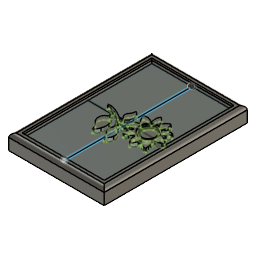
Test 2 tournesol (Autodesk Fusion 360 design; units mm, degrees)
part number: 2026-04-24-15-50-29-841
Autodesk Fusion 360 part; units mm, degrees
box "BoitePrimitive1" add length 75 width 50 height 8 placed x (0, -1, 0) y (1, 0, 0) z (0, 0, 1) at (0, 0, 0)
sketch "Esquisse2" plane through (0, 0, 8) normal (0, 0, 1) x (-1, 0, 0)
  line L0 (0, 75) -> (-50, 75)
  line L1 (-50, 75) -> (-50, 0)
  line L2 (-50, 0) -> (0, 0)
  line L3 (0, 0) -> (0, 75)
  line L4 (-4.0213, 75) -> (-4.0213, 0)
  line L5 (0, 4.0248) -> (-50, 4.0248)
  line L6 (-46.0257, 0) -> (-46.0257, 75)
  line L7 (-50, 70.9503) -> (0, 70.9503)
  point P0 (-4.0213, 70.9503)
  point P1 (-46.0257, 70.9503)
  point P2 (-46.0257, 4.0248)
  point P3 (-4.0213, 4.0248)
  constraint coincident L0 L4.start
  constraint coincident L2 L4.end
  constraint perpendicular L2 L4
  constraint coincident L3 L5.start
  constraint coincident L1 L5.end
  constraint perpendicular L1 L5
  constraint coincident L2 L6.start
  constraint coincident L0 L6.end
  constraint perpendicular L0 L6
  constraint coincident L1 L7.start
  constraint coincident L3 L7.end
  constraint perpendicular L3 L7
  constraint coincident L7 P0
  constraint coincident L4 P0
  constraint coincident L6 P1
  constraint coincident L7 P1
  constraint coincident L6 P2
  constraint coincident L5 P2
  constraint coincident L5 P3
  constraint coincident L4 P3
extrude "Extrusion1" cut sketch "Esquisse2" against normal blind 2 contours L4 L5 L6 L7
fillet "Congé1" radius 2 4 edges at (25, 0, 8) (50, -37.5, 8) (25, -75, 8) (0, -37.5, 8)
fillet "Congé2" radius 0.5 4 edges at (25.0235, -4.0248, 8) (46.0257, -37.4876, 8) (25.0235, -70.9503, 8) (4.0213, -37.4876, 8)
sketch "Esquisse3" plane through (0, 0, 6) normal (0, 0, 1) x (-1, 0, 0)
  line L0 (-46.0257, 4.0248) -> (-4.0213, 4.0248)
  line L1 (-4.0213, 4.0248) -> (-4.0213, 70.9503)
  line L2 (-4.0213, 70.9503) -> (-46.0257, 70.9503)
  line L3 (-46.0257, 70.9503) -> (-46.0257, 4.0248)
  line L4 (-25.0235, 4.0248) -> (-25.0235, 70.9503)
  line L5 (-4.0213, 37.4876) -> (-46.0257, 37.4876)
  line L6 (-25.4937, 4.0248) -> (-25.4937, 70.9503)
  line L7 (-24.5013, 4.0248) -> (-24.5013, 70.9503)
  spline S0 degree 3 poles (-13.2534, 35.811) (-13.4823, 35.5969) (-15.4305, 35.9038) (-16.7842, 36.3672) knots 0 0 0 0 1 1 1 1
  spline S1 degree 3 poles (-16.7842, 36.3672) (-17.692, 36.678) (-19.587, 37.5732) (-20.54, 38.1415) knots 0 0 0 0 1 1 1 1
  spline S2 degree 3 poles (-20.54, 38.1415) (-21.6835, 38.8234) (-22.4957, 39.02) (-23.1364, 38.7701) knots 0 0 0 0 1 1 1 1
  spline S3 degree 3 poles (-23.1364, 38.7701) (-23.4033, 38.666) (-23.4058, 38.6626) (-23.3252, 38.5087) knots 0 0 0 0 1 1 1 1
  spline S4 degree 3 poles (-23.3252, 38.5087) (-23.2804, 38.4229) (-23.0386, 38.1071) (-22.7879, 37.807) knots 0 0 0 0 1 1 1 1
  spline S5 degree 3 poles (-22.7879, 37.807) (-22.5373, 37.5068) (-22.2677, 37.1329) (-22.1889, 36.9761) knots 0 0 0 0 1 1 1 1
  spline S6 degree 3 poles (-22.1889, 36.9761) (-21.8625, 36.3265) (-21.9778, 35.5072) (-22.4877, 34.8523) knots 0 0 0 0 1 1 1 1
  spline S7 degree 3 poles (-22.4877, 34.8523) (-23.2739, 33.8426) (-23.3292, 33.7283) (-23.4429, 32.8776) knots 0 0 0 0 1 1 1 1
  spline S8 degree 3 poles (-23.4429, 32.8776) (-23.5405, 32.1474) (-23.5565, 32.0964) (-23.7039, 32.0427) knots 0 0 0 0 1 1 1 1
  spline S9 degree 3 poles (-23.7039, 32.0427) (-23.8507, 31.9893) (-23.8907, 32.0077) (-24.3137, 32.3228) knots 0 0 0 0 1 1 1 1
  spline S10 degree 3 poles (-24.3137, 32.3228) (-25.4296, 33.1541) (-26.1693, 34.5636) (-26.1594, 35.8399) knots 0 0 0 0 1 1 1 1
  spline S11 degree 3 poles (-26.1594, 35.8399) (-26.1548, 36.4262) (-25.9675, 37.136) (-25.7116, 37.5369) knots 0 0 0 0 1 1 1 1
  spline S12 degree 3 poles (-25.7116, 37.5369) (-25.4079, 38.0125) (-24.7673, 38.5558) (-24.2808, 38.7503) knots 0 0 0 0 1 1 1 1
  spline S13 degree 3 poles (-24.2808, 38.7503) (-24.0446, 38.8447) (-23.717, 39) (-23.5527, 39.0955) knots 0 0 0 0 1 1 1 1
  spline S14 degree 3 poles (-23.5527, 39.0955) (-23.1919, 39.3052) (-22.7265, 39.3936) (-22.2525, 39.3422) knots 0 0 0 0 1 1 1 1
  spline S15 degree 3 poles (-22.2525, 39.3422) (-22.0589, 39.3212) (-21.9143, 39.3361) (-21.9312, 39.3753) knots 0 0 0 0 1 1 1 1
  spline S16 degree 3 poles (-21.9312, 39.3753) (-22.0154, 39.5708) (-23.3025, 40.3477) (-24.3294, 40.823) knots 0 0 0 0 1 1 1 1
  spline S17 degree 3 poles (-24.3294, 40.823) (-25.2456, 41.2471) (-25.5259, 41.3479) (-26.188, 41.4917) knots 0 0 0 0 1 1 1 1
  spline S18 degree 3 poles (-26.188, 41.4917) (-27.4482, 41.7653) (-28.566, 41.7741) (-29.7633, 41.5197) knots 0 0 0 0 1 1 1 1
  spline S19 degree 3 poles (-29.7633, 41.5197) (-30.0286, 41.4634) (-30.3169, 41.4134) (-30.4041, 41.4085) knots 0 0 0 0 1 1 1 1
  spline S20 degree 3 poles (-30.4041, 41.4085) (-30.609, 41.3973) (-31.0876, 40.728) (-31.0212, 40.5455) knots 0 0 0 0 1 1 1 1
  spline S21 degree 3 poles (-31.0212, 40.5455) (-31.0135, 40.5245) (-30.8196, 40.5139) (-30.5901, 40.522) knots 0 0 0 0 1 1 1 1
  spline S22 degree 3 poles (-30.5901, 40.522) (-30.3607, 40.5301) (-30.1121, 40.5389) (-30.0376, 40.5415) knots 0 0 0 0 1 1 1 1
  spline S23 degree 3 poles (-30.0376, 40.5415) (-29.7942, 40.5502) (-29.0635, 40.4545) (-28.6359, 40.3579) knots 0 0 0 0 1 1 1 1
  spline S24 degree 3 poles (-28.6359, 40.3579) (-28.2014, 40.2597) (-26.5617, 39.5188) (-26.2895, 39.2977) knots 0 0 0 0 1 1 1 1
  spline S25 degree 3 poles (-26.2895, 39.2977) (-26.1466, 39.1816) (-26.1483, 39.1565) (-26.3238, 38.7809) knots 0 0 0 0 1 1 1 1
  spline S26 degree 3 poles (-26.3238, 38.7809) (-26.4253, 38.5638) (-26.5807, 38.3308) (-26.6691, 38.2631) knots 0 0 0 0 1 1 1 1
  spline S27 degree 3 poles (-26.6691, 38.2631) (-26.7575, 38.1954) (-26.8893, 38.0659) (-26.9619, 37.9752) knots 0 0 0 0 1 1 1 1
  spline S28 degree 3 poles (-26.9619, 37.9752) (-27.0345, 37.8846) (-27.2951, 37.6725) (-27.5409, 37.5038) knots 0 0 0 0 1 1 1 1
  spline S29 degree 3 poles (-27.5409, 37.5038) (-27.7867, 37.3352) (-27.9969, 37.1778) (-28.008, 37.154) knots 0 0 0 0 1 1 1 1
  spline S30 degree 3 poles (-28.008, 37.154) (-28.019, 37.1303) (-28.1248, 37.0882) (-28.243, 37.0605) knots 0 0 0 0 1 1 1 1
  spline S31 degree 3 poles (-28.243, 37.0605) (-28.3612, 37.0328) (-28.4608, 36.9866) (-28.4644, 36.9579) knots 0 0 0 0 1 1 1 1
  spline S32 degree 3 poles (-28.4644, 36.9579) (-28.4754, 36.8699) (-29.5329, 36.455) (-30.0799, 36.3241) knots 0 0 0 0 1 1 1 1
  spline S33 degree 3 poles (-30.0799, 36.3241) (-30.6696, 36.1831) (-30.6481, 36.1277) (-29.8052, 35.6164) knots 0 0 0 0 1 1 1 1
  spline S34 degree 3 poles (-29.8052, 35.6164) (-29.5603, 35.4678) (-29.0495, 35.0412) (-29.0277, 34.9671) knots 0 0 0 0 1 1 1 1
  spline S35 degree 3 poles (-29.0277, 34.9671) (-29.0195, 34.9392) (-28.9051, 34.8066) (-28.7734, 34.6724) knots 0 0 0 0 1 1 1 1
  spline S36 degree 3 poles (-28.7734, 34.6724) (-28.6418, 34.5382) (-28.4108, 34.2239) (-28.2601, 33.974) knots 0 0 0 0 1 1 1 1
  spline S37 degree 3 poles (-28.2601, 33.974) (-28.1093, 33.724) (-27.9401, 33.4561) (-27.8839, 33.3787) knots 0 0 0 0 1 1 1 1
  spline S38 degree 3 poles (-27.8839, 33.3787) (-27.726, 33.1609) (-27.3691, 32.205) (-27.3593, 31.9737) knots 0 0 0 0 1 1 1 1
  spline S39 degree 3 poles (-27.3593, 31.9737) (-27.3513, 31.7837) (-27.3694, 31.7607) (-27.5812, 31.6926) knots 0 0 0 0 1 1 1 1
  spline S40 degree 3 poles (-27.5812, 31.6926) (-27.9245, 31.5821) (-28.9894, 31.5368) (-29.0506, 31.6301) knots 0 0 0 0 1 1 1 1
  spline S41 degree 3 poles (-29.0506, 31.6301) (-29.0818, 31.6777) (-29.0997, 31.6761) (-29.0938, 31.6263) knots 0 0 0 0 1 1 1 1
  spline S42 degree 3 poles (-29.0938, 31.6263) (-29.0845, 31.5476) (-29.2191, 31.5418) (-29.7301, 31.5993) knots 0 0 0 0 1 1 1 1
  spline S43 degree 3 poles (-29.7301, 31.5993) (-30.2675, 31.6598) (-31.202, 32.0241) (-31.7872, 32.4011) knots 0 0 0 0 1 1 1 1
  spline S44 degree 3 poles (-31.7872, 32.4011) (-32.3647, 32.7733) (-32.5127, 32.7687) (-32.378, 32.3826) knots 0 0 0 0 1 1 1 1
  spline S45 degree 3 poles (-32.378, 32.3826) (-32.144, 31.7115) (-32.0367, 31.2191) (-32.1072, 31.1394) knots 0 0 0 0 1 1 1 1
  spline S46 degree 3 poles (-32.1072, 31.1394) (-32.1271, 31.1169) (-32.1155, 31.0855) (-32.0814, 31.0695) knots 0 0 0 0 1 1 1 1
  spline S47 degree 3 poles (-32.0814, 31.0695) (-32.0008, 31.032) (-31.9788, 30.42) (-32.0551, 30.3394) knots 0 0 0 0 1 1 1 1
  spline S48 degree 3 poles (-32.0551, 30.3394) (-32.0873, 30.3055) (-32.0912, 30.2083) (-32.0638, 30.1235) knots 0 0 0 0 1 1 1 1
  spline S49 degree 3 poles (-32.0638, 30.1235) (-31.9808, 29.8664) (-32.1499, 29.0508) (-32.402, 28.4923) knots 0 0 0 0 1 1 1 1
  line L8 (-32.402, 28.4923) -> (-32.6368, 27.972)
  line L9 (-32.6368, 27.972) -> (-32.889, 28.0653)
  spline S50 degree 3 poles (-32.889, 28.0653) (-33.5693, 28.3168) (-34.7121, 29.5435) (-35.0582, 30.3936) knots 0 0 0 0 1 1 1 1
  spline S51 degree 3 poles (-35.0582, 30.3936) (-35.1169, 30.5376) (-35.1832, 30.664) (-35.2056, 30.6745) knots 0 0 0 0 1 1 1 1
  spline S52 degree 3 poles (-35.2056, 30.6745) (-35.228, 30.6849) (-35.3089, 30.8654) (-35.3854, 31.0754) knots 0 0 0 0 1 1 1 1
  spline S53 degree 3 poles (-35.3854, 31.0754) (-35.5823, 31.6167) (-35.6909, 31.5992) (-35.9797, 30.98) knots 0 0 0 0 1 1 1 1
  spline S54 degree 3 poles (-35.9797, 30.98) (-36.2419, 30.4177) (-36.7819, 29.6388) (-37.0124, 29.4904) knots 0 0 0 0 1 1 1 1
  spline S55 degree 3 poles (-37.0124, 29.4904) (-37.0979, 29.4354) (-37.2222, 29.3289) (-37.2887, 29.2538) knots 0 0 0 0 1 1 1 1
  spline S56 degree 3 poles (-37.2887, 29.2538) (-37.6098, 28.891) (-38.5441, 28.4985) (-38.7142, 28.6549) knots 0 0 0 0 1 1 1 1
  spline S57 degree 3 poles (-38.7142, 28.6549) (-38.9378, 28.8604) (-39.3649, 30.5048) (-39.2556, 30.7392) knots 0 0 0 0 1 1 1 1
  spline S58 degree 3 poles (-39.2556, 30.7392) (-39.2355, 30.7823) (-39.2322, 30.8567) (-39.2483, 30.9045) knots 0 0 0 0 1 1 1 1
  spline S59 degree 3 poles (-39.2483, 30.9045) (-39.3222, 31.1242) (-39.1568, 32.136) (-38.9653, 32.6357) knots 0 0 0 0 1 1 1 1
  spline S60 degree 3 poles (-38.9653, 32.6357) (-38.8412, 32.9594) (-38.7843, 33.1977) (-38.8218, 33.2365) knots 0 0 0 0 1 1 1 1
  spline S61 degree 3 poles (-38.8218, 33.2365) (-38.8559, 33.2719) (-39.0406, 33.2194) (-39.232, 33.1199) knots 0 0 0 0 1 1 1 1
  spline S62 degree 3 poles (-39.232, 33.1199) (-39.7819, 32.8342) (-40.7036, 32.4666) (-40.7804, 32.5024) knots 0 0 0 0 1 1 1 1
  spline S63 degree 3 poles (-40.7804, 32.5024) (-40.8189, 32.5204) (-40.9701, 32.4965) (-41.1165, 32.4494) knots 0 0 0 0 1 1 1 1
  spline S64 degree 3 poles (-41.1165, 32.4494) (-41.2628, 32.4023) (-41.4412, 32.381) (-41.5129, 32.402) knots 0 0 0 0 1 1 1 1
  spline S65 degree 3 poles (-41.5129, 32.402) (-41.5845, 32.423) (-41.7466, 32.4211) (-41.8729, 32.3978) knots 0 0 0 0 1 1 1 1
  spline S66 degree 3 poles (-41.8729, 32.3978) (-42.0991, 32.356) (-42.7741, 32.3853) (-42.8984, 32.4422) knots 0 0 0 0 1 1 1 1
  spline S67 degree 3 poles (-42.8984, 32.4422) (-42.9333, 32.4582) (-43.103, 32.4929) (-43.2753, 32.5192) knots 0 0 0 0 1 1 1 1
  spline S68 degree 3 poles (-43.2753, 32.5192) (-43.4477, 32.5456) (-43.5965, 32.5888) (-43.6061, 32.6152) knots 0 0 0 0 1 1 1 1
  spline S69 degree 3 poles (-43.6061, 32.6152) (-43.6157, 32.6416) (-43.5775, 32.8004) (-43.5211, 32.9682) knots 0 0 0 0 1 1 1 1
  spline S70 degree 3 poles (-43.5211, 32.9682) (-43.4648, 33.136) (-43.4363, 33.3001) (-43.4578, 33.3328) knots 0 0 0 0 1 1 1 1
  spline S71 degree 3 poles (-43.4578, 33.3328) (-43.5679, 33.5006) (-42.8835, 34.6096) (-42.4069, 35.0356) knots 0 0 0 0 1 1 1 1
  spline S72 degree 3 poles (-42.4069, 35.0356) (-42.3289, 35.1054) (-42.2167, 35.2093) (-42.1574, 35.2665) knots 0 0 0 0 1 1 1 1
  spline S73 degree 3 poles (-42.1574, 35.2665) (-41.9396, 35.4771) (-41.515, 35.8235) (-41.2709, 35.9898) knots 0 0 0 0 1 1 1 1
  spline S74 degree 3 poles (-41.2709, 35.9898) (-41.1329, 36.0838) (-41.0298, 36.1876) (-41.0417, 36.2205) knots 0 0 0 0 1 1 1 1
  spline S75 degree 3 poles (-41.0417, 36.2205) (-41.0537, 36.2533) (-41.3097, 36.3325) (-41.6106, 36.3964) knots 0 0 0 0 1 1 1 1
  spline S76 degree 3 poles (-41.6106, 36.3964) (-42.2495, 36.532) (-44.1971, 37.3516) (-44.1452, 37.4629) knots 0 0 0 0 1 1 1 1
  spline S77 degree 3 poles (-44.1452, 37.4629) (-44.1282, 37.4994) (-44.1783, 37.5596) (-44.2565, 37.5965) knots 0 0 0 0 1 1 1 1
  spline S78 degree 3 poles (-44.2565, 37.5965) (-44.7398, 37.8247) (-45.5611, 38.8988) (-45.442, 39.1468) knots 0 0 0 0 1 1 1 1
  spline S79 degree 3 poles (-45.442, 39.1468) (-45.416, 39.201) (-45.1665, 39.4036) (-44.8877, 39.5972) knots 0 0 0 0 1 1 1 1
  spline S80 degree 3 poles (-44.8877, 39.5972) (-44.171, 40.0948) (-43.0417, 40.4235) (-41.9841, 40.4426) knots 0 0 0 0 1 1 1 1
  spline S81 degree 3 poles (-41.9841, 40.4426) (-41.4011, 40.4531) (-41.0901, 40.4323) (-40.8392, 40.3662) knots 0 0 0 0 1 1 1 1
  spline S82 degree 3 poles (-40.8392, 40.3662) (-40.5079, 40.2788) (-40.4417, 40.448) (-40.7154, 40.6824) knots 0 0 0 0 1 1 1 1
  spline S83 degree 3 poles (-40.7154, 40.6824) (-40.8213, 40.7732) (-40.9144, 40.8709) (-40.9223, 40.8995) knots 0 0 0 0 1 1 1 1
  spline S84 degree 3 poles (-40.9223, 40.8995) (-40.9301, 40.9282) (-41.0402, 41.0645) (-41.1668, 41.2025) knots 0 0 0 0 1 1 1 1
  spline S85 degree 3 poles (-41.1668, 41.2025) (-41.846, 41.9422) (-41.9475, 42.1105) (-42.3027, 43.0836) knots 0 0 0 0 1 1 1 1
  spline S86 degree 3 poles (-42.3027, 43.0836) (-42.5, 43.6242) (-42.6896, 44.2707) (-42.7241, 44.5202) knots 0 0 0 0 1 1 1 1
  spline S87 degree 3 poles (-42.7241, 44.5202) (-42.8006, 45.0733) (-42.7973, 45.6931) (-42.7175, 45.7454) knots 0 0 0 0 1 1 1 1
  spline S88 degree 3 poles (-42.7175, 45.7454) (-42.6852, 45.7666) (-42.6848, 45.839) (-42.7166, 45.9063) knots 0 0 0 0 1 1 1 1
  spline S89 degree 3 poles (-42.7166, 45.9063) (-42.85, 46.1884) (-42.6393, 46.2534) (-41.9946, 46.1291) knots 0 0 0 0 1 1 1 1
  spline S90 degree 3 poles (-41.9946, 46.1291) (-41.0884, 45.9544) (-39.3037, 45.008) (-39.1519, 44.6217) knots 0 0 0 0 1 1 1 1
  spline S91 degree 3 poles (-39.1519, 44.6217) (-39.1334, 44.5748) (-39.0609, 44.507) (-38.9906, 44.4712) knots 0 0 0 0 1 1 1 1
  spline S92 degree 3 poles (-38.9906, 44.4712) (-38.9203, 44.4353) (-38.8024, 44.312) (-38.7287, 44.1972) knots 0 0 0 0 1 1 1 1
  spline S93 degree 3 poles (-38.7287, 44.1972) (-38.6549, 44.0823) (-38.5155, 43.8972) (-38.4189, 43.7858) knots 0 0 0 0 1 1 1 1
  spline S94 degree 3 poles (-38.4189, 43.7858) (-38.3224, 43.6744) (-38.2314, 43.5275) (-38.2168, 43.4594) knots 0 0 0 0 1 1 1 1
  spline S95 degree 3 poles (-38.2168, 43.4594) (-38.1941, 43.3539) (-38.1667, 43.3404) (-38.0301, 43.3673) knots 0 0 0 0 1 1 1 1
  spline S96 degree 3 poles (-38.0301, 43.3673) (-37.8739, 43.3982) (-37.8701, 43.4072) (-37.876, 43.7373) knots 0 0 0 0 1 1 1 1
  spline S97 degree 3 poles (-37.876, 43.7373) (-37.8793, 43.9234) (-37.8712, 44.1487) (-37.858, 44.238) knots 0 0 0 0 1 1 1 1
  spline S98 degree 3 poles (-37.858, 44.238) (-37.8448, 44.3274) (-37.8607, 44.4129) (-37.8932, 44.428) knots 0 0 0 0 1 1 1 1
  spline S99 degree 3 poles (-37.8932, 44.428) (-37.9257, 44.4432) (-37.9182, 44.5288) (-37.8765, 44.6182) knots 0 0 0 0 1 1 1 1
  spline S100 degree 3 poles (-37.8765, 44.6182) (-37.8347, 44.7077) (-37.8042, 44.8459) (-37.8086, 44.9254) knots 0 0 0 0 1 1 1 1
  spline S101 degree 3 poles (-37.8086, 44.9254) (-37.8419, 45.5301) (-36.7505, 47.5481) (-36.2727, 47.7651) knots 0 0 0 0 1 1 1 1
  spline S102 degree 3 poles (-36.2727, 47.7651) (-36.1351, 47.8276) (-36.0983, 47.7955) (-35.6678, 47.2364) knots 0 0 0 0 1 1 1 1
  spline S103 degree 3 poles (-35.6678, 47.2364) (-35.4157, 46.909) (-35.1343, 46.4982) (-35.0426, 46.3235) knots 0 0 0 0 1 1 1 1
  spline S104 degree 3 poles (-35.0426, 46.3235) (-34.8169, 45.8938) (-34.3795, 44.6037) (-34.3712, 44.3433) knots 0 0 0 0 1 1 1 1
  spline S105 degree 3 poles (-34.3712, 44.3433) (-34.3675, 44.2276) (-34.3457, 44.0419) (-34.3227, 43.9308) knots 0 0 0 0 1 1 1 1
  spline S106 degree 3 poles (-34.3227, 43.9308) (-34.2997, 43.8196) (-34.3082, 43.7107) (-34.3416, 43.6888) knots 0 0 0 0 1 1 1 1
  spline S107 degree 3 poles (-34.3416, 43.6888) (-34.3749, 43.6669) (-34.374, 43.6358) (-34.3394, 43.6197) knots 0 0 0 0 1 1 1 1
  spline S108 degree 3 poles (-34.3394, 43.6197) (-34.3048, 43.6035) (-34.2864, 43.5168) (-34.2985, 43.427) knots 0 0 0 0 1 1 1 1
  spline S109 degree 3 poles (-34.2985, 43.427) (-34.3194, 43.2723) (-34.2707, 43.1285) (-34.1828, 43.0849) knots 0 0 0 0 1 1 1 1
  spline S110 degree 3 poles (-34.1828, 43.0849) (-34.1609, 43.074) (-34.0244, 43.1918) (-33.8795, 43.3466) knots 0 0 0 0 1 1 1 1
  spline S111 degree 3 poles (-33.8795, 43.3466) (-33.4099, 43.8482) (-32.761, 44.3431) (-32.3394, 44.521) knots 0 0 0 0 1 1 1 1
  spline S112 degree 3 poles (-32.3394, 44.521) (-31.5239, 44.8653) (-31.0317, 45.0047) (-30.6142, 45.0099) knots 0 0 0 0 1 1 1 1
  spline S113 degree 3 poles (-30.6142, 45.0099) (-30.4754, 45.0116) (-30.3507, 45.0371) (-30.337, 45.0665) knots 0 0 0 0 1 1 1 1
  spline S114 degree 3 poles (-30.337, 45.0665) (-30.3232, 45.096) (-30.2293, 45.1041) (-30.1282, 45.0847) knots 0 0 0 0 1 1 1 1
  spline S115 degree 3 poles (-30.1282, 45.0847) (-29.9883, 45.0577) (-29.9279, 44.9978) (-29.8752, 44.8336) knots 0 0 0 0 1 1 1 1
  spline S116 degree 3 poles (-29.8752, 44.8336) (-29.8101, 44.6313) (-29.8055, 43.8896) (-29.8684, 43.7546) knots 0 0 0 0 1 1 1 1
  spline S117 degree 3 poles (-29.8684, 43.7546) (-29.8841, 43.721) (-29.8991, 43.585) (-29.9017, 43.4525) knots 0 0 0 0 1 1 1 1
  spline S118 degree 3 poles (-29.9017, 43.4525) (-29.9075, 43.156) (-30.1378, 42.3498) (-30.2683, 42.1691) knots 0 0 0 0 1 1 1 1
  spline S119 degree 3 poles (-30.2683, 42.1691) (-30.339, 42.0712) (-30.338, 42.0589) (-30.2645, 42.1223) knots 0 0 0 0 1 1 1 1
  spline S120 degree 3 poles (-30.2645, 42.1223) (-30.1202, 42.2468) (-28.6077, 42.4639) (-27.8847, 42.4638) knots 0 0 0 0 1 1 1 1
  spline S121 degree 3 poles (-27.8847, 42.4638) (-26.5747, 42.4636) (-25.3812, 42.2066) (-24.153, 41.66) knots 0 0 0 0 1 1 1 1
  spline S122 degree 3 poles (-24.153, 41.66) (-23.7233, 41.4688) (-23.3756, 41.3209) (-23.3803, 41.3314) knots 0 0 0 0 1 1 1 1
  spline S123 degree 3 poles (-23.3803, 41.3314) (-23.3851, 41.3419) (-23.6044, 41.6333) (-23.8676, 41.9789) knots 0 0 0 0 1 1 1 1
  spline S124 degree 3 poles (-23.8676, 41.9789) (-24.4105, 42.6919) (-24.776, 43.2115) (-25.1764, 43.8398) knots 0 0 0 0 1 1 1 1
  spline S125 degree 3 poles (-25.1764, 43.8398) (-25.4526, 44.2731) (-25.4538, 44.2741) (-25.9084, 44.4213) knots 0 0 0 0 1 1 1 1
  spline S126 degree 3 poles (-25.9084, 44.4213) (-28.0505, 45.1152) (-29.3455, 47.0599) (-29.0245, 49.1009) knots 0 0 0 0 1 1 1 1
  spline S127 degree 3 poles (-29.0245, 49.1009) (-28.8533, 50.1898) (-27.8181, 51.7262) (-27.0983, 51.9598) knots 0 0 0 0 1 1 1 1
  spline S128 degree 3 poles (-27.0983, 51.9598) (-26.8061, 52.0547) (-26.6706, 51.9349) (-26.6129, 51.5309) knots 0 0 0 0 1 1 1 1
  spline S129 degree 3 poles (-26.6129, 51.5309) (-26.3954, 50.0065) (-26.3241, 49.8576) (-25.5392, 49.2862) knots 0 0 0 0 1 1 1 1
  spline S130 degree 3 poles (-25.5392, 49.2862) (-25.2597, 49.0827) (-24.9073, 48.7718) (-24.7562, 48.5954) knots 0 0 0 0 1 1 1 1
  spline S131 degree 3 poles (-24.7562, 48.5954) (-24.0941, 47.8222) (-23.9321, 46.4994) (-24.3614, 45.3721) knots 0 0 0 0 1 1 1 1
  spline S132 degree 3 poles (-24.3614, 45.3721) (-24.7516, 44.3473) (-24.7634, 44.1368) (-24.4572, 43.6587) knots 0 0 0 0 1 1 1 1
  spline S133 degree 3 poles (-24.4572, 43.6587) (-23.8591, 42.725) (-22.6996, 41.2924) (-21.9924, 40.6135) knots 0 0 0 0 1 1 1 1
  spline S134 degree 3 poles (-21.9924, 40.6135) (-21.4133, 40.0574) (-20.583, 39.3928) (-19.7759, 38.8393) knots 0 0 0 0 1 1 1 1
  spline S135 degree 3 poles (-19.7759, 38.8393) (-19.0695, 38.3549) (-17.4282, 37.4633) (-17.2758, 37.4812) knots 0 0 0 0 1 1 1 1
  spline S136 degree 3 poles (-17.2758, 37.4812) (-17.2307, 37.4866) (-17.3297, 37.6547) (-17.4959, 37.8548) knots 0 0 0 0 1 1 1 1
  spline S137 degree 3 poles (-17.4959, 37.8548) (-18.015, 38.4804) (-18.2862, 38.9904) (-18.7031, 40.1251) knots 0 0 0 0 1 1 1 1
  line L10 (-18.7031, 40.1251) -> (-19.1067, 41.2235)
  line L11 (-19.1067, 41.2235) -> (-19.6293, 41.4672)
  spline S138 degree 3 poles (-19.6293, 41.4672) (-20.3283, 41.7931) (-20.673, 42.0514) (-21.1286, 42.5904) knots 0 0 0 0 1 1 1 1
  spline S139 degree 3 poles (-21.1286, 42.5904) (-21.6381, 43.1933) (-21.913, 43.7466) (-22.1142, 44.5744) knots 0 0 0 0 1 1 1 1
  spline S140 degree 3 poles (-22.1142, 44.5744) (-22.4217, 45.8391) (-22.3518, 47.1) (-21.8953, 48.5284) knots 0 0 0 0 1 1 1 1
  spline S141 degree 3 poles (-21.8953, 48.5284) (-21.6107, 49.4189) (-21.1341, 50.2818) (-20.5844, 50.902) knots 0 0 0 0 1 1 1 1
  spline S142 degree 3 poles (-20.5844, 50.902) (-20.0867, 51.4635) (-19.9909, 51.4385) (-19.8691, 50.715) knots 0 0 0 0 1 1 1 1
  spline S143 degree 3 poles (-19.8691, 50.715) (-19.6899, 49.65) (-19.0311, 48.4666) (-18.2424, 47.7927) knots 0 0 0 0 1 1 1 1
  spline S144 degree 3 poles (-18.2424, 47.7927) (-18.0836, 47.6569) (-17.8229, 47.4349) (-17.6631, 47.2992) knots 0 0 0 0 1 1 1 1
  spline S145 degree 3 poles (-17.6631, 47.2992) (-16.7092, 46.4893) (-16.1045, 44.9895) (-16.2776, 43.8634) knots 0 0 0 0 1 1 1 1
  spline S146 degree 3 poles (-16.2776, 43.8634) (-16.3772, 43.2163) (-16.6322, 42.6324) (-16.9957, 42.2198) knots 0 0 0 0 1 1 1 1
  spline S147 degree 3 poles (-16.9957, 42.2198) (-17.3535, 41.8136) (-17.8056, 41.4676) (-18.1752, 41.3172) knots 0 0 0 0 1 1 1 1
  spline S148 degree 3 poles (-18.1752, 41.3172) (-18.4961, 41.1866) (-18.502, 41.033) (-18.2153, 40.2643) knots 0 0 0 0 1 1 1 1
  spline S149 degree 3 poles (-18.2153, 40.2643) (-17.9503, 39.5537) (-17.5736, 38.8543) (-17.2007, 38.3802) knots 0 0 0 0 1 1 1 1
  spline S150 degree 3 poles (-17.2007, 38.3802) (-16.6751, 37.712) (-16.4161, 37.49) (-15.748, 37.135) knots 0 0 0 0 1 1 1 1
  spline S151 degree 3 poles (-15.748, 37.135) (-15.0734, 36.7765) (-15.0616, 36.7734) (-13.4665, 36.5329) knots 0 0 0 0 1 1 1 1
  spline S152 degree 3 poles (-13.4665, 36.5329) (-13.2378, 36.4985) (-13.1885, 36.4671) (-13.1244, 36.315) knots 0 0 0 0 1 1 1 1
  spline S153 degree 3 poles (-13.1244, 36.315) (-13.0529, 36.1454) (-13.1024, 35.9522) (-13.2534, 35.811) knots 0 0 0 0 1 1 1 1
  spline S154 degree 3 poles (-33.9037, 41.9547) (-31.956, 40.6715) (-30.674, 38.4784) (-31.1092, 36.1366) knots 0 0 0 0 1 1 1 1
  spline S155 degree 3 poles (-31.1092, 36.1366) (-31.4082, 34.5276) (-32.5787, 33.0509) (-34.1371, 32.4684) knots 0 0 0 0 1 1 1 1
  spline S156 degree 3 poles (-34.1371, 32.4684) (-35.5216, 31.9346) (-37.1176, 32.3047) (-38.2793, 33.1781) knots 0 0 0 0 1 1 1 1
  spline S157 degree 3 poles (-38.2793, 33.1781) (-39.7153, 34.1748) (-40.7575, 35.8134) (-40.794, 37.5891) knots 0 0 0 0 1 1 1 1
  spline S158 degree 3 poles (-40.794, 37.5891) (-40.8321, 39.2392) (-40.1629, 41.0134) (-38.7252, 41.9244) knots 0 0 0 0 1 1 1 1
  spline S159 degree 3 poles (-38.7252, 41.9244) (-37.2802, 43.1464) (-35.344, 42.9036) (-33.9037, 41.9547) knots 0 0 0 0 1 1 1 1
  spline S160 degree 3 poles (-34.3105, 41.053) (-32.2758, 39.9217) (-31.7326, 38.107) (-32.0752, 36.3991) knots 0 0 0 0 1 1 1 1
  spline S161 degree 3 poles (-32.0752, 36.3991) (-32.3271, 35.1436) (-33.0526, 34.0078) (-34.4973, 33.4649) knots 0 0 0 0 1 1 1 1
  spline S162 degree 3 poles (-34.4973, 33.4649) (-35.6083, 33.0474) (-36.8814, 33.3339) (-37.8106, 34.0326) knots 0 0 0 0 1 1 1 1
  spline S163 degree 3 poles (-37.8106, 34.0326) (-38.9593, 34.8298) (-39.793, 36.1406) (-39.8221, 37.5609) knots 0 0 0 0 1 1 1 1
  spline S164 degree 3 poles (-39.8221, 37.5609) (-39.8526, 38.8809) (-39.3174, 40.3) (-38.1673, 41.0288) knots 0 0 0 0 1 1 1 1
  spline S165 degree 3 poles (-38.1673, 41.0288) (-37.0486, 41.6752) (-36.0001, 41.9924) (-34.3105, 41.053) knots 0 0 0 0 1 1 1 1
  spline S166 degree 3 poles (-34.5021, 40.6284) (-33.1293, 39.8001) (-32.3227, 38.1274) (-32.5302, 36.5227) knots 0 0 0 0 1 1 1 1
  spline S167 degree 3 poles (-32.5302, 36.5227) (-32.6761, 35.3943) (-33.606, 34.3805) (-34.6669, 33.9342) knots 0 0 0 0 1 1 1 1
  spline S168 degree 3 poles (-34.6669, 33.9342) (-35.5159, 33.577) (-36.7847, 33.8401) (-37.5996, 34.4629) knots 0 0 0 0 1 1 1 1
  spline S169 degree 3 poles (-37.5996, 34.4629) (-38.548, 35.1879) (-39.255, 36.31) (-39.3644, 37.5477) knots 0 0 0 0 1 1 1 1
  spline S170 degree 3 poles (-39.3644, 37.5477) (-39.4508, 38.5257) (-38.9243, 39.9228) (-37.9045, 40.607) knots 0 0 0 0 1 1 1 1
  spline S171 degree 3 poles (-37.9045, 40.607) (-36.8954, 41.2517) (-35.5241, 41.2338) (-34.5021, 40.6284) knots 0 0 0 0 1 1 1 1
  constraint midpoint L0 L4.start
  constraint midpoint L2 L4.end
  constraint midpoint L1 L5.start
  constraint midpoint L3 L5.end
  constraint coincident L0 L6.start
  constraint perpendicular L2 L6
  constraint coincident L0 L7.start
  constraint perpendicular L2 L7
extrude "Extrusion2" add sketch "Esquisse3" along normal blind 2 contours L5 L6 S10 S11 | L4 L5 L6 S10 | L5 L6 S17 S18 S19 S20 S21 S22 S23 S24 S25 S26 S27 S28 S29 S77 S78 S79 S80 S81 S82 S83 S84 S85 S86 S87 S88 S89 S90 S91 S92 S93 S94 S95 S96 S97 S98 S99 S100 S101 S102 S103 S104 S105 S106 S107 S108 S109 S110 S111 S112 S113 S114 S115 S116 S117 S118 S119 S120 S121 S154 S157 S158 S159 | L5 S29 S30 S31 S32 S33 S34 S35 S36 S37 S38 S39 S40 S41 S42 S43 S44 S45 S46 S47 S48 S49 L8 L9 S50 S51 S52 S53 S54 S55 S56 S57 S58 S59 S60 S61 S62 S63 S64 S65 S66 S67 S68 S69 S70 S71 S72 S73 S74 S75 S76 S77 S154 S155 S156 S157 | L4 L5 L7 S10 | L4 L5 L6 S12 | L5 L6 S11 S12 | L5 L7 S5 S6 S7 S8 S9 S10 | L4 L5 L7 S12 | L4 L6 S124 S125 S130 | L6 S125 S126 S127 S128 S129 S130 | L5 L7 S1 S2 S3 S4 S5 S12 S13 S14 S15 S16 S17 S121 S122 S123 S124 S132 S133 S134 S135 | L4 L6 S17 S121 | L4 L7 S124 S130 S131 S132 | L5 S0 S1 S135 S136 S150 S151 S152 S153 | L5 S136 S137 L10 L11 S138 S139 S140 S141 S142 S143 S144 S145 S146 S147 S148 S149 S150 | L4 L7 S17 S121 | L7 S131 S132
extrude "Extrusion3" add sketch "Esquisse3" along normal blind 1.5 contours L5 S154 S157 S158 S159 S160 S163 S164 S165 | L5 S154 S155 S156 S157 S160 S161 S162 S163
extrude "Extrusion4" add sketch "Esquisse3" along normal blind 1 contours L5 S160 S163 S164 S165 S166 S169 S170 S171 | L5 S160 S161 S162 S163 S166 S167 S168 S169
extrude "Extrusion5" add sketch "Esquisse3" along normal blind 0.5 contours L5 S166 S169 S170 S171 | L5 S166 S167 S168 S169
